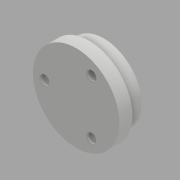
# Autodesk Inventor part: Arm - slew column B
Saved by Autodesk Inventor 2017 (Build 210142000, 142)
## iProperties
Created: 2017-06-18
Part Number: Arm - slew column B
Material: Generic
Document SubType Name: Modeling
Designer: Ali
Density: 1 g/cm^3
Appearance: Default
Author: Ali
Autodesk Inventor part; units mm, degrees
ref_plane "YZ Plane" through (0, 0, 0) normal (1, 0, 0) x (0, 1, 0)
ref_plane "XZ Plane" through (0, 0, 0) normal (0, 1, 0) x (-1, 0, 0)
ref_plane "XY Plane" through (0, 0, 0) normal (0, 0, 1) x (1, 0, 0)
sketch "Sketch1" plane through (0, 0, 0) normal (0, 1, 0) x (-1, 0, 0)
  circle A0 centre (0, 0) radius 20
  dimension "d0" = 40
  constraints: 1 centre point, 1 coincident
  measures "d0" diameter of A0
extrude "Extrusion1" add sketch "Sketch1" along normal blind 6
sketch "Sketch2" plane through (0, 6, 0) normal (0, 1, 0) x (1, 0, 0)
  circle A0 centre (0, 0) radius 17.5
  dimension "d3" = 35
  constraints: 1 centre point, 1 coincident
  measures "d3" diameter of A0
extrude "Extrusion2" add sketch "Sketch2" along normal blind 6.8
sketch "Sketch3" plane through (0, 12.8, 0) normal (0, 1, 0) x (1, 0, 0)
  circle A0 centre (0, 0) radius 14.5 construction
  line L0 (0, 0) -> (-14.5, 0) construction
  point P0 (7.25, -12.5574)
  point P1 (7.25, 12.5574)
  dimension "d6" = 29
  dimension "d9" = 360
  constraints: 2 end point, 1 coincident, 1 horizontal, 1 horizontal alignment, 6 other
hole "Hole1" at (-14.5, 12.8, 0) at (7.25, 12.8, 12.5574) at (7.25, 12.8, -12.5574) direction (0, -1, 0) diameter 4.3 end through all
body "Solid1"
